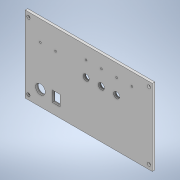
# Autodesk Inventor part: Box Top
Saved by Autodesk Inventor 2022 (Build 260153000, 153)
## iProperties
Created: 2021-07-04
Part Number: Box Top
Material: Generic
Document SubType Name: Modeling
Designer: Matthijs
Density: 1 g/cm^3
Appearance: Default
Author: Matthijs
Autodesk Inventor part; units mm, degrees
ref_plane "YZ Plane" through (0, 0, 0) normal (1, 0, 0) x (0, 1, 0)
ref_plane "XZ Plane" through (0, 0, 0) normal (0, 1, 0) x (-1, 0, 0)
ref_plane "XY Plane" through (0, 0, 0) normal (0, 0, 1) x (1, 0, 0)
sketch "Sketch1" plane through (0, 0, 0) normal (0, 0, 1) x (1, 0, 0)
  line L0 (125, -75) -> (-125, -75)
  line L1 (-125, -75) -> (-125, 75)
  line L2 (-125, 75) -> (125, 75)
  line L3 (125, 75) -> (125, -75)
  line L4 (125, -75) -> (-125, 75) construction
  line L5 (-125, -75) -> (125, 75) construction
  point P0 (0, 0)
  dimension "d0" = 250
  dimension "d1" = 150
  constraints: 12 end point, 2 midpoint, 2 parallel, 1 horizontal, 1 perpendicular
  measures "d0" distance of L1.end L2.end
  measures "d1" distance of L0.end L1.end
extrude "Extrusion1" add sketch "Sketch1" along normal blind 5
sketch "Sketch2" plane through (0, 0, 5) normal (0, 0, 1) x (1, 0, 0)
  line L0 (-125, -75) -> (125, -75) projected
  line L1 (-125, -75) -> (-112, -75)
  line L2 (-112, -75) -> (-112, -57)
  line L3 (-112, -57) -> (-125, -57)
  line L4 (-125, -57) -> (-125, -75)
  line L5 (125, -75) -> (125, 75) projected
  line L6 (125, -75) -> (112, -75)
  line L7 (112, -75) -> (112, -57)
  line L8 (112, -57) -> (125, -57)
  line L9 (125, -57) -> (125, -75)
  line L10 (125, 75) -> (-125, 75) projected
  line L11 (-125, 75) -> (-112, 75)
  line L12 (-112, 75) -> (-112, 57)
  line L13 (-112, 57) -> (-125, 57)
  line L14 (-125, 57) -> (-125, 75)
  line L15 (125, 75) -> (112, 75)
  line L16 (112, 75) -> (112, 57)
  line L17 (112, 57) -> (125, 57)
  line L18 (125, 57) -> (125, 75)
  line L19 (-125, 75) -> (-112, 57)
  line L20 (-112, 75) -> (-125, 57)
  line L21 (112, 75) -> (125, 57)
  line L22 (125, 57) -> (125, 75)
  line L23 (112, 57) -> (125, 75)
  line L24 (125, -75) -> (112, -57)
  line L25 (125, -57) -> (112, -75)
  line L26 (-125, -57) -> (-112, -75)
  line L27 (-125, 75) -> (-125, -75) projected
  line L28 (-112, -57) -> (-125, -75)
  point P0 (0, 0)
  point P1 (-118.5, -66)
  point P2 (-118.5, 66)
  point P3 (118.5, 66)
  point P4 (118.5, -66)
  dimension "d4" = 13
  dimension "d5" = 18
  dimension "d6" = 13
  dimension "d7" = 18
  dimension "d8" = 13
  dimension "d9" = 18
  dimension "d10" = 13
  dimension "d11" = 18
  constraints: 50 end point, 9 parallel, 4 horizontal, 4 midpoint, 4 perpendicular, 2 point on line, 1 vertical
  measures "d4" distance of L3.end L2.end
  measures "d5" distance of L2.end L1.end
  measures "d6" distance of L7.end L8.end
  measures "d7" distance of L6.end L7.end
  measures "d8" distance of L12.end L13.end
  measures "d9" distance of L11.end L12.end
  measures "d10" distance of L17.end L16.end
  measures "d11" distance of L16.end L15.end
hole "Hole1" at (-118.5, -66, 5) at (118.5, 66, 5) at (118.5, -66, 5) at (-118.5, 66, 5) direction (0, 0, -1) diameter 3.4 end through all counterbore diameter 6.5 counterbore depth 3.4 clearance for "Socket Head Cap Screw DIN EN ISO 4762" size "M3" standard "DIN"
sketch "Sketch34" plane through (0, 0, 5) normal (0, 0, 1) x (1, 0, 0)
  circle A0 centre (-95, 35) radius 1.7
  line L0 (125, 75) -> (-125, 75) projected
  line L1 (-125, 75) -> (-125, -75) projected
  point P0 (0, 0)
  dimension "d166" = 3.4
  dimension "d169" = 40
  dimension "d170" = 30
  constraints: 1 centre point
  measures "d166" diameter of A0
  measures "d169" distance from line of L0 A0.centre
  measures "d170" distance from line of L1 A0.centre
extrude "ToggleswitchWithCap1" cut sketch "Sketch34" against normal blind 10
sketch "Sketch36" plane through (0, 0, 5) normal (0, 0, 1) x (1, 0, 0)
  circle A0 centre (-65, 35) radius 1.7
  line L0 (125, 75) -> (-125, 75) projected
  line L1 (-125, 75) -> (-125, -75) projected
  point P0 (0, 0)
  dimension "d171" = 3.4
  dimension "d172" = 40
  dimension "d173" = 60
  constraints: 1 centre point
  measures "d171" diameter of A0
  measures "d172" distance from line of L0 A0.centre
  measures "d173" distance from line of L1 A0.centre
extrude "ToggleSwitchWithCap2" cut sketch "Sketch36" against normal through all
sketch "Sketch38" plane through (0, 0, 5) normal (0, 0, 1) x (1, 0, 0)
  line L0 (-71.5, -34.5) -> (-56.5, -34.5)
  line L1 (-56.5, -34.5) -> (-56.5, -55.5)
  line L2 (-56.5, -55.5) -> (-71.5, -55.5)
  line L3 (-71.5, -55.5) -> (-71.5, -34.5)
  line L4 (125, 75) -> (-125, 75) projected
  line L5 (-125, 75) -> (-125, -75) projected
  point P0 (0, 0)
  dimension "d181" = 15
  dimension "d182" = 21
  dimension "d185" = 109.5
  dimension "d186" = 53.5
  constraints: 8 end point, 2 parallel, 1 horizontal, 1 perpendicular
  measures "d181" distance of L1.end L2.end
  measures "d182" distance of L0.end L1.end
  measures "d185" distance between parallel lines of L4 L0
  measures "d186" distance between parallel lines of L5 L3
extrude "OnOffToggle" cut sketch "Sketch38" against normal through all
sketch "Sketch17" plane through (0, 0, 5) normal (0, 0, 1) x (1, 0, 0)
  circle A0 centre (-95, -45) radius 9.5
  line L0 (125, 75) -> (-125, 75) projected
  line L1 (-125, 75) -> (-125, -75) projected
  point P0 (0, 0)
  point P1 (-104.4472, 75)
  point P2 (-85.5528, 75)
  dimension "d81" = 19
  dimension "d82" = 120
  dimension "d83" = 30
  constraints: 1 centre point
  measures "d81" diameter of A0
  measures "d82" distance from line of L0 A0.centre
  measures "d83" distance from line of L1 A0.centre
extrude "KeySwitch" cut sketch "Sketch17" against normal through all
sketch "Sketch18" plane through (0, 0, 5) normal (0, 0, 1) x (1, 0, 0)
  circle A0 centre (-5, 50) radius 1.7
  line L0 (-125, 75) -> (-125, -75) projected
  line L1 (125, 75) -> (-125, 75) projected
  point P0 (0, 0)
  dimension "d86" = 3.4
  dimension "d98" = 120
  dimension "d99" = 25
  constraints: 1 centre point
  measures "d86" diameter of A0
  measures "d98" distance from line of L0 A0.centre
  measures "d99" distance from line of L1 A0.centre
extrude "Toggleswitch1" cut sketch "Sketch18" against normal through all
sketch "Sketch19" plane through (0, 0, 5) normal (0, 0, 1) x (1, 0, 0)
  circle A0 centre (25, 50) radius 1.7
  line L0 (125, 75) -> (-125, 75) projected
  line L1 (-125, 75) -> (-125, -75) projected
  point P0 (0, 0)
  dimension "d89" = 3.4
  dimension "d100" = 25
  dimension "d101" = 150
  constraints: 1 centre point
  measures "d89" diameter of A0
  measures "d100" distance from line of L0 A0.centre
  measures "d101" distance from line of L1 A0.centre
extrude "Toggleswitch2" cut sketch "Sketch19" against normal through all
sketch "Sketch20" plane through (0, 0, 5) normal (0, 0, 1) x (1, 0, 0)
  circle A0 centre (55, 50) radius 1.7
  line L0 (125, 75) -> (-125, 75) projected
  line L1 (-125, 75) -> (-125, -75) projected
  point P0 (0, 0)
  dimension "d92" = 3.4
  dimension "d102" = 25
  dimension "d103" = 180
  constraints: 1 centre point
  measures "d92" diameter of A0
  measures "d102" distance from line of L0 A0.centre
  measures "d103" distance from line of L1 A0.centre
extrude "Toggleswitch3" cut sketch "Sketch20" against normal through all
sketch "Sketch21" plane through (0, 0, 5) normal (0, 0, 1) x (1, 0, 0)
  circle A0 centre (85, 50) radius 1.7
  line L0 (125, 75) -> (-125, 75) projected
  line L1 (-125, 75) -> (-125, -75) projected
  point P0 (0, 0)
  dimension "d95" = 3.4
  dimension "d104" = 25
  dimension "d105" = 210
  constraints: 1 centre point
  measures "d95" diameter of A0
  measures "d104" distance from line of L0 A0.centre
  measures "d105" distance from line of L1 A0.centre
extrude "Toggleswitch4" cut sketch "Sketch21" against normal through all
sketch "Sketch22" plane through (0, 0, 5) normal (0, 0, 1) x (1, 0, 0)
  circle A0 centre (-5, 20) radius 6
  line L0 (-125, 75) -> (-125, -75) projected
  line L1 (125, 75) -> (-125, 75) projected
  point P0 (0, 0)
  dimension "d106" = 12
  dimension "d109" = 120
  dimension "d110" = 55
  constraints: 1 centre point
  measures "d106" diameter of A0
  measures "d109" distance from line of L0 A0.centre
  measures "d110" distance from line of L1 A0.centre
extrude "ButtonBlack1" cut sketch "Sketch22" against normal through all
sketch "Sketch23" plane through (0, 0, 5) normal (0, 0, 1) x (1, 0, 0)
  circle A0 centre (25, 20) radius 6
  line L0 (125, 75) -> (-125, 75) projected
  line L1 (-125, 75) -> (-125, -75) projected
  point P0 (0, 0)
  dimension "d111" = 12
  dimension "d114" = 55
  dimension "d115" = 150
  constraints: 1 centre point
  measures "d111" diameter of A0
  measures "d114" distance from line of L0 A0.centre
  measures "d115" distance from line of L1 A0.centre
extrude "ButtonBlack2" cut sketch "Sketch23" against normal through all
sketch "Sketch24" plane through (0, 0, 5) normal (0, 0, 1) x (1, 0, 0)
  circle A0 centre (55, 20) radius 6
  line L0 (125, 75) -> (-125, 75) projected
  line L1 (-125, 75) -> (-125, -75) projected
  point P0 (0, 0)
  dimension "d116" = 12
  dimension "d117" = 55
  dimension "d118" = 180
  constraints: 1 centre point
  measures "d116" diameter of A0
  measures "d117" distance from line of L0 A0.centre
  measures "d118" distance from line of L1 A0.centre
extrude "ButtonBlack3" cut sketch "Sketch24" against normal through all
sketch "Sketch25" plane through (0, 0, 5) normal (0, 0, 1) x (1, 0, 0)
  circle A0 centre (85, 20) radius 6
  line L0 (125, 75) -> (-125, 75) projected
  line L1 (-125, 75) -> (-125, -75) projected
  point P0 (0, 0)
  dimension "d121" = 12
  dimension "d122" = 55
  dimension "d123" = 210
  constraints: 1 centre point
  measures "d121" diameter of A0
  measures "d122" distance from line of L0 A0.centre
  measures "d123" distance from line of L1 A0.centre
sketch "Sketch26" plane through (0, 0, 5) normal (0, 0, 1) x (1, 0, 0)
  circle A0 centre (-5, -10) radius 6
  line L0 (-125, 75) -> (-125, -75) projected
  line L1 (125, 75) -> (-125, 75) projected
  point P0 (0, 0)
  dimension "d126" = 12
  dimension "d127" = 120
  dimension "d128" = 85
  constraints: 1 centre point
  measures "d126" diameter of A0
  measures "d127" distance from line of L0 A0.centre
  measures "d128" distance from line of L1 A0.centre
sketch "Sketch27" plane through (0, 0, 5) normal (0, 0, 1) x (1, 0, 0)
  circle A0 centre (25, -10) radius 6
  line L0 (125, 75) -> (-125, 75) projected
  line L1 (-125, 75) -> (-125, -75) projected
  point P0 (0, 0)
  dimension "d131" = 12
  dimension "d132" = 85
  dimension "d133" = 150
  constraints: 1 centre point
  measures "d131" diameter of A0
  measures "d132" distance from line of L0 A0.centre
  measures "d133" distance from line of L1 A0.centre
sketch "Sketch28" plane through (0, 0, 5) normal (0, 0, 1) x (1, 0, 0)
  circle A0 centre (55, -10) radius 6
  line L0 (125, 75) -> (-125, 75) projected
  line L1 (-125, 75) -> (-125, -75) projected
  point P0 (0, 0)
  dimension "d136" = 12
  dimension "d137" = 85
  dimension "d138" = 180
  constraints: 1 centre point
  measures "d136" diameter of A0
  measures "d137" distance from line of L0 A0.centre
  measures "d138" distance from line of L1 A0.centre
sketch "Sketch29" plane through (0, 0, 5) normal (0, 0, 1) x (1, 0, 0)
  circle A0 centre (85, -10) radius 6
  line L0 (125, 75) -> (-125, 75) projected
  line L1 (-125, 75) -> (-125, -75) projected
  point P0 (0, 0)
  dimension "d141" = 12
  dimension "d142" = 85
  dimension "d143" = 210
  constraints: 1 centre point
  measures "d141" diameter of A0
  measures "d142" distance from line of L0 A0.centre
  measures "d143" distance from line of L1 A0.centre
sketch "Sketch30" plane through (0, 0, 5) normal (0, 0, 1) x (1, 0, 0)
  circle A0 centre (-5, -45) radius 10
  line L0 (125, 75) -> (-125, 75) projected
  line L1 (-125, 75) -> (-125, -75) projected
  point P0 (0, 0)
  dimension "d146" = 20
  dimension "d147" = 120
  dimension "d148" = 120
  constraints: 1 centre point
  measures "d146" diameter of A0
  measures "d147" distance from line of L0 A0.centre
  measures "d148" distance from line of L1 A0.centre
sketch "Sketch31" plane through (0, 0, 5) normal (0, 0, 1) x (1, 0, 0)
  circle A0 centre (25, -45) radius 10
  line L0 (125, 75) -> (-125, 75) projected
  line L1 (-125, 75) -> (-125, -75) projected
  point P0 (0, 0)
  dimension "d151" = 20
  dimension "d152" = 120
  dimension "d153" = 150
  constraints: 1 centre point
  measures "d151" diameter of A0
  measures "d152" distance from line of L0 A0.centre
  measures "d153" distance from line of L1 A0.centre
sketch "Sketch32" plane through (0, 0, 5) normal (0, 0, 1) x (1, 0, 0)
  circle A0 centre (55, -45) radius 10
  line L0 (125, 75) -> (-125, 75) projected
  line L1 (-125, 75) -> (-125, -75) projected
  point P0 (0, 0)
  dimension "d156" = 20
  dimension "d157" = 120
  dimension "d158" = 180
  constraints: 1 centre point
  measures "d156" diameter of A0
  measures "d157" distance from line of L0 A0.centre
  measures "d158" distance from line of L1 A0.centre
sketch "Sketch33" plane through (0, 0, 5) normal (0, 0, 1) x (1, 0, 0)
  circle A0 centre (85, -45) radius 10
  line L0 (125, 75) -> (-125, 75) projected
  line L1 (-125, 75) -> (-125, -75) projected
  point P0 (0, 0)
  dimension "d161" = 20
  dimension "d162" = 120
  dimension "d163" = 210
  constraints: 1 centre point
  measures "d161" diameter of A0
  measures "d162" distance from line of L0 A0.centre
  measures "d163" distance from line of L1 A0.centre
body "Solid1"
